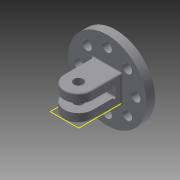
# Autodesk Inventor part: right_angle_holder
Saved by Autodesk Inventor 2013 (Build 170138000, 138)
## iProperties
Created: 2013-03-18
Part Number: right_angle_holder
Material: Generic
Document SubType Name: Modeling
Designer: Mahisorn
Density: 1 g/cm^3
Author: Mahisorn
Autodesk Inventor part; units mm, degrees
ref_plane "YZ Plane" through (0, 0, 0) normal (1, 0, 0) x (0, 1, 0)
ref_plane "XZ Plane" through (0, 0, 0) normal (0, 1, 0) x (-1, 0, 0)
ref_plane "XY Plane" through (0, 0, 0) normal (0, 0, 1) x (1, 0, 0)
sketch "Sketch1" plane through (0, 0, 0) normal (0, 1, 0) x (-1, 0, 0)
  circle A0 centre (0, 0) radius 27.5
  dimension "d0" = 55
  constraints: 1 centre point, 1 coincident
  measures "d0" diameter of A0
extrude "Extrusion1" add sketch "Sketch1" along normal blind 6
sketch "Sketch2" plane through (0, 6, 0) normal (0, 1, 0) x (1, 0, 0)
  circle A0 centre (0, 0) radius 27.5 projected
  point P0 (20, 0)
  point P1 (14.1421, 14.1421)
  point P2 (0, 20)
  point P3 (-14.1421, 14.1421)
  point P4 (-20, 0)
  point P5 (-14.1421, -14.1421)
  point P6 (0, -20)
  point P7 (14.1421, -14.1421)
  dimension "d3" = 20
  dimension "d6" = 360
  constraints: 9 other
  measures "d3" distance of A0.centre point (20, 0)
hole "Hole1" at (20, 6, 0) at (14.1421, 6, -14.1421) at (0, 6, -20) at (-14.1421, 6, -14.1421) at (-20, 6, 0) at (-14.1421, 6, 14.1421) at (0, 6, 20) at (14.1421, 6, 14.1421) direction (0, -1, 0) diameter 6.6 depth 8 tip angle 118 clearance for "Flat Head Machine Screw" size "M6" standard "Ansi Metric M Profile"
sketch "Sketch8" plane through (0, 6, 0) normal (0, 1, 0) x (1, 0, 0)
  circle A0 centre (0, 0) radius 27.5 projected
  line L0 (-9, 10) -> (9, 10)
  line L1 (9, 10) -> (9, -10)
  line L2 (9, -10) -> (-9, -10)
  line L3 (-9, -10) -> (-9, 10)
  point P0 (0, 10)
  point P1 (9, 0)
  dimension "d28" = 18
  dimension "d30" = 20
  constraints: 8 end point, 2 midpoint, 2 parallel, 1 horizontal, 1 horizontal alignment, 1 perpendicular, 1 vertical alignment
  measures "d28" distance of L0.start L0.end
  measures "d30" distance of L2.end L0.start
extrude "Extrusion3" add sketch "Sketch8" along normal blind 30 contours L0 L1 L2 L3
sketch "Sketch9" plane through (0, 36, 0) normal (0, 1, 0) x (1, 0, 0)
  line L0 (9, 10) -> (-9, 10) projected
  line L1 (-9, -10) -> (9, -10) projected
  line L2 (-3, 10) -> (3, 10)
  line L3 (3, 10) -> (3, -10)
  line L4 (3, -10) -> (-3, -10)
  line L5 (-3, -10) -> (-3, 10)
  point P0 (0, 0)
  point P1 (0, 10)
  point P2 (0, 10)
  dimension "d54" = 6
  constraints: 8 end point, 2 midpoint, 2 parallel, 2 point on line, 2 vertical alignment, 1 horizontal, 1 perpendicular
  measures "d54" distance between parallel lines of L3 L5
sketch "Sketch10" plane through (9, 6, 10) normal (1, 0, 0) x (0, 0, -1)
  line L0 (20, 0) -> (0, 0) projected
  line L1 (20, 0) -> (20, 30) projected
  line L2 (0, 30) -> (20, 30) projected
  line L3 (0, 0) -> (0, 30) projected
  point P0 (10, -6)
fillet "Fillet2" radius 10 2 edges at (0, 36, 10) (0, 36, -10)
sketch "Sketch11" plane through (9, 6, 10) normal (1, 0, 0) x (0, 0, -1)
  arc A0 (20, 20) -> (0, 20) centre (10, 20) ccw projected
  point P0 (10, -6)
  constraints: 1 coincident
hole "Hole3" at (9, 26, 0) direction (-1, 0, 0) diameter 6.6 end through all clearance for "Flat Head Machine Screw" size "M6" standard "Ansi Metric M Profile"
extrude "Extrusion4" cut sketch "Sketch9" against normal blind 25
sketch "Sketch12" plane through (-9, 6, 10) normal (0, 0, 1) x (1, 0, 0)
  line L0 (6, 5) -> (6, 20) projected
  line L1 (12, 20) -> (12, 5) projected
  line L2 (12, 5) -> (6, 5) projected
  arc A0 (6, 6) -> (6, 4) centre (6, 5) ccw
  line L3 (6, 5) -> (6, 4) construction
  line L4 (6, 5) -> (6, 6) construction
  arc A1 (12, 4) -> (12, 6) centre (12, 5) ccw
  line L5 (12, 5) -> (12, 4) construction
  line L6 (12, 5) -> (12, 6) construction
  line L7 (6, 6) -> (12, 6)
  line L8 (6, 4) -> (12, 4)
  point P0 (9, -6)
  dimension "d45" = 1
  dimension "d46" = 180
  dimension "d47" = 1
  dimension "d48" = 180
  constraints: 12 end point, 4 point on circle, 2 centre point, 2 coincident, 2 point on line
  measures "d45" radius of A0
  measures "d46" angle of L4 L3
  measures "d47" radius of A1
  measures "d48" angle of L6 L5
extrude "Extrusion5" cut sketch "Sketch12" against normal through all contours L2 L1 A1 L8 A0 L0
fillet "Fillet3" radius 1 4 edges at (0, 6, 10) (-9, 6, 0) (9, 6, 0) (0, 6, -10)
fillet "Fillet4" radius 1 10 edges at (9, 33.0711, -7.0711) (9, 16.5001, -10) (9.2929, 6.2929, -10.2929) (9.2929, 6.2929, 10.2929) (9, 16.5001, 10) (-9, 33.0711, -7.0711) (-9, 16.5001, 10) (-9.2929, 6.2929, 10.2929) (-9.2929, 6.2929, -10.2929) (-9, 16.5001, -10)
body "Solid1"
